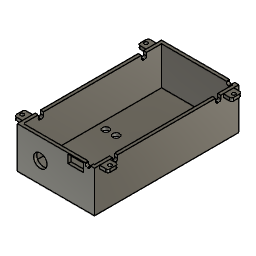
Cover_V3 (Autodesk Fusion 360 design; units mm, degrees)
part number: 2025-10-18-14-32-01-691
Autodesk Fusion 360 part; units mm, degrees
sketch "Sketch1" plane through (0, 0, 0) normal (0, 0, 1) x (1, 0, 0)
  line L0 (0, 0) -> (69, 0)
  line L1 (69, 0) -> (69, 140)
  line L2 (69, 140) -> (0, 140)
  line L3 (0, 140) -> (0, 0)
  line L4 (0, 140) -> (-3, 140)
  line L5 (-3, 140) -> (-3, 0)
  line L6 (-3, 0) -> (0, 0)
  line L7 (0, 0) -> (0, 140)
  line L8 (69, 140) -> (72, 140)
  line L9 (72, 140) -> (72, 0)
  line L10 (72, 0) -> (69, 0)
  line L11 (69, 0) -> (69, 140)
  line L12 (34.5, 140) -> (34.5, 0) construction
  line L13 (25, 0) -> (44, 0)
  line L14 (34.5, 2) -> (34.5, 0) construction
  circle A0 centre (8, 75) radius 3.275
  circle A1 centre (60, 60) radius 6
  circle A2 centre (18, 75) radius 3.275
  line L15 (1.1966, 84.5922) -> (38.7187, 84.5357) construction
  line L16 (38.7187, 84.5357) -> (38.7111, 79.5066) construction
  line L17 (38.7111, 79.5066) -> (1.189, 79.563) construction
  line L18 (1.189, 79.563) -> (1.1966, 84.5922) construction
  circle A3 centre (60, 40) radius 3.5
  line L19 (69, 3) -> (0, 3)
  line L20 (69, 137) -> (0, 137)
  circle A4 centre (77, 130) radius 1.7
  line L21 (72, 140) -> (112, 140) construction
  line L22 (72, 125) -> (78, 125)
  line L23 (80, 127) -> (80, 133)
  line L24 (78, 135) -> (72, 135)
  line L25 (72, 135) -> (72, 125)
  circle A5 centre (77, 10) radius 1.7
  line L26 (72, 0) -> (100, 0) construction
  line L27 (72, 5) -> (78, 5)
  line L28 (80, 7) -> (80, 13)
  line L29 (78, 15) -> (72, 15)
  line L30 (72, 15) -> (72, 5)
  circle A6 centre (-8, 10) radius 1.7
  line L31 (-3, 0) -> (-18, 0) construction
  line L32 (-3, 15) -> (-9, 15)
  line L33 (-11, 13) -> (-11, 7)
  line L34 (-9, 5) -> (-3, 5)
  line L35 (-3, 5) -> (-3, 15)
  line L36 (-3, 140) -> (-16, 140) construction
  circle A7 centre (-8, 130) radius 1.7
  line L37 (-3, 135) -> (-9, 135)
  line L38 (-11, 133) -> (-11, 127)
  line L39 (-9, 125) -> (-3, 125)
  line L40 (-3, 125) -> (-3, 135) construction
  arc A8 (-11, 127) -> (-9, 125) centre (-9, 127) ccw
  arc A9 (-9, 135) -> (-11, 133) centre (-9, 133) ccw
  arc A10 (-9, 15) -> (-11, 13) centre (-9, 13) ccw
  arc A11 (-11, 7) -> (-9, 5) centre (-9, 7) ccw
  arc A12 (80, 13) -> (78, 15) centre (78, 13) ccw
  arc A13 (78, 5) -> (80, 7) centre (78, 7) ccw
  arc A14 (78, 125) -> (80, 127) centre (78, 127) ccw
  arc A15 (80, 133) -> (78, 135) centre (78, 133) ccw
  point P0 (-11, 15)
  point P1 (-11, 135)
  dimension "d1" = 140
  dimension "d3" = 3
  dimension "d4" = 3
  dimension "d30" = 75
  dimension "d35" = 6.55
  dimension "d36" = 65
  dimension "d37" = 12
  dimension "d38" = 60
  dimension "d40" = 6.55
  dimension "d41" = 10
  dimension "d42" = 3.5
  dimension "d46" = 7
  dimension "d47" = 40
  dimension "d48" = 3
  dimension "d49" = 3
  dimension "d64" = 3.4
  dimension "d65" = 5
  dimension "d66" = 10
  dimension "d67" = 8
  dimension "d68" = 10
  dimension "d69" = 5
  dimension "d70" = 3.4
  dimension "d71" = 5
  dimension "d72" = 10
  dimension "d73" = 10
  dimension "d74" = 5
  dimension "d75" = 8
  dimension "d76" = 3.4
  dimension "d77" = 5
  dimension "d78" = 10
  dimension "d79" = 8
  dimension "d80" = 10
  dimension "d81" = 5
  dimension "d82" = 3.4
  dimension "d83" = 5
  dimension "d84" = 10
  dimension "d85" = 8
  dimension "d86" = 10
  dimension "d87" = 5
  dimension "d88" = 2
  dimension "d89" = 2
  dimension "d90" = 2
  dimension "d91" = 2
  dimension "d92" = 2
  dimension "d93" = 2
  dimension "d94" = 2
  dimension "d95" = 2
  text T0 "CELL GPS\n" font "Arial" height 3.5 align left top in box 37.5222 x 5.0292 at (1.1966, 84.5922) x (0.999999, -0.001504) y (-0.001504, -0.999999) spacing 1 kerned
  constraint horizontal L0
  constraint vertical L1
  constraint horizontal L2
  constraint vertical L3
  constraint coincident L0.start L3.end
  constraint horizontal L4
  constraint vertical L5
  constraint horizontal L6
  constraint vertical L7
  constraint horizontal L8
  constraint vertical L9
  constraint horizontal L10
  constraint vertical L11
  constraint midpoint L2 L12.start
  constraint midpoint L0 L12.end
  constraint horizontal L13
  constraint coincident L0 L13.start
  constraint midpoint L13 L12.end
  constraint coincident L12 L14.start
  constraint coincident L1 L19.start
  constraint coincident L3 L19.end
  constraint perpendicular L3 L19
  constraint coincident L1 L20.start
  constraint perpendicular L1 L20
  constraint perpendicular L9 L21
  constraint horizontal L22
  constraint vertical L23
  constraint horizontal L24
  constraint vertical L25
  constraint coincident L9 L22.start
  constraint perpendicular L9 L26
  constraint horizontal L27
  constraint vertical L28
  constraint horizontal L29
  constraint vertical L30
  constraint coincident L9 L27.start
  constraint perpendicular L5 L31
  constraint horizontal L32
  constraint vertical L33
  constraint horizontal L34
  constraint vertical L35
  constraint coincident L5 L32.start
  constraint perpendicular L5 L36
  constraint horizontal L37
  constraint vertical L38
  constraint horizontal L39
  constraint vertical L40
  constraint coincident L5 L37.start
  constraint tangent L38 A8
  constraint tangent L39 A8
  constraint coincident P1 L37
  constraint coincident P1 L38
  constraint tangent L37 A9
  constraint tangent L38 A9
  constraint coincident P0 L32
  constraint coincident P0 L33
  constraint tangent L32 A10
  constraint tangent L33 A10
  constraint tangent L33 A11
  constraint tangent L34 A11
  constraint tangent L28 A12
  constraint tangent L29 A12
  constraint tangent L27 A13
  constraint tangent L28 A13
  constraint tangent L22 A14
  constraint tangent L23 A14
  constraint tangent L23 A15
  constraint tangent L24 A15
  measures "d1" distance of L0.start L2.end
  measures "d3" distance of L5 L7
  measures "d4" distance of L9 L11
  measures "d30" distance of L5 L9
  measures "d35" diameter of A0
  measures "d36" distance of L2 A0.centre
  measures "d37" diameter of A1
  measures "d38" distance of L0 A1.centre
  measures "d40" diameter of A2
  measures "d41" distance of A0.centre A2.centre
  measures "d46" diameter of A3
  measures "d47" distance of L0 A3.centre
  measures "d48" distance of L13 L19
  measures "d49" distance of L2 L20
  measures "d64" diameter of A4
  measures "d65" distance of L9 A4.centre
  measures "d66" distance of A4.centre L21
  measures "d67" distance of L23 L25
  measures "d68" distance of L22 L24
  measures "d69" distance of L21 L24
  measures "d70" diameter of A5
  measures "d71" distance of L9 A5.centre
  measures "d72" distance of A5.centre L26
  measures "d73" distance of L27 L29
  measures "d74" distance of L26 L27
  measures "d75" distance of L9 L28
  measures "d76" diameter of A6
  measures "d77" distance of L5 A6.centre
  measures "d78" distance of A6.centre L31
  measures "d79" distance of L32.start P0
  measures "d80" distance of L32.start L34.end
  measures "d81" distance of L31 L34
  measures "d82" diameter of A7
  measures "d83" distance of L5 A7.centre
  measures "d84" distance of L36 A7.centre
  measures "d85" distance of L37.start P1
  measures "d86" distance of L37.start L39.end
  measures "d87" distance of L36 L37
  measures "d88" radius of A8
  measures "d89" radius of A9
  measures "d90" radius of A10
  measures "d91" radius of A11
  measures "d92" radius of A12
  measures "d93" radius of A13
  measures "d94" radius of A14
  measures "d95" radius of A15
extrude "Extrude1" add sketch "Sketch1" along normal blind 3 contours L0 L1 L3 L7 L11 L13 L19 | L1 L3 L7 L11 L19 L20 | L1 L2 L3 L7 L11 L20 makes body 1
extrude "Extrude2" add sketch "Sketch1" along normal blind 40 contours L0 L1 L3 L7 L11 L13 L19 | L3 L4 L5 L6 L7 L35 | L1 L2 L3 L7 L11 L20 | L1 L8 L9 L10 L11 L25 L30 bodies 1
sketch "Sketch3" plane through (72, 0, 0) normal (1, 0, 0) x (0, 1, 0)
  line L0 (0, 0) -> (140, 0)
  line L1 (140, 0) -> (140, 40)
  line L2 (140, 40) -> (0, 40)
  line L3 (0, 40) -> (0, 0)
  line L4 (140, 0) -> (0, 0)
  line L5 (70, 40) -> (70, 0) construction
  line L6 (17.5, 40) -> (22.5, 40)
  line L7 (22.5, 40) -> (22.5, 37)
  line L8 (20.5, 35) -> (19.5, 35)
  line L9 (17.5, 37) -> (17.5, 40)
  arc A0 (17.5, 37) -> (19.5, 35) centre (19.5, 37) ccw
  arc A1 (20.5, 35) -> (22.5, 37) centre (20.5, 37) ccw
  line L10 (20, 40) -> (20, 35) construction
  line L11 (117.5, 40) -> (122.5, 40)
  line L12 (122.5, 40) -> (122.5, 37)
  line L13 (120.5, 35) -> (119.5, 35)
  line L14 (117.5, 37) -> (117.5, 40)
  arc A2 (117.5, 37) -> (119.5, 35) centre (119.5, 37) ccw
  arc A3 (120.5, 35) -> (122.5, 37) centre (120.5, 37) ccw
  line L15 (120, 35) -> (120, 40) construction
  point P0 (17.5, 35)
  point P1 (117.5, 35)
  dimension "d18" = 5
  dimension "d19" = 5
  dimension "d20" = 2
  dimension "d21" = 2
  dimension "d23" = 5
  dimension "d24" = 2
  dimension "d25" = 2
  dimension "d26" = 5
  dimension "d27" = 100
  constraint midpoint L2 L5.start
  constraint midpoint L4 L5.end
  constraint horizontal L6
  constraint vertical L7
  constraint horizontal L8
  constraint vertical L9
  constraint coincident L2 L6.start
  constraint coincident P0 L8
  constraint coincident P0 L9
  constraint tangent L8 A0
  constraint tangent L9 A0
  constraint tangent L7 A1
  constraint tangent L8 A1
  constraint midpoint L6 L10.start
  constraint midpoint L8 L10.end
  constraint horizontal L11
  constraint vertical L12
  constraint horizontal L13
  constraint vertical L14
  constraint coincident L2 L11.start
  constraint coincident P1 L13
  constraint coincident P1 L14
  constraint tangent L13 A2
  constraint tangent L14 A2
  constraint tangent L12 A3
  constraint tangent L13 A3
  constraint midpoint L13 L15.start
  constraint midpoint L11 L15.end
  constraint symmetric L5 L10 L15
  measures "d18" distance of L6.start P0
  measures "d19" distance of L7 L9
  measures "d20" radius of A0
  measures "d21" radius of A1
  measures "d23" distance of L12 L14
  measures "d24" radius of A2
  measures "d25" radius of A3
  measures "d26" distance of L11 L13
  measures "d27" distance of L10 L15
extrude "Extrude3" cut sketch "Sketch3" along normal mid plane 200 contours L2 L6 L7 L8 L9 A0 A1 | L2 L11 L12 L13 L14 A2 A3 bodies 1
extrude "Extrude4" cut sketch "Sketch1" along normal blind 1 text T0 bodies 1
sketch "Sketch4" plane through (0, 0, 0) normal (0, -1, 0) x (1, 0, 0)
  line L0 (-3, 0) -> (72, 0)
  line L1 (72, 0) -> (72, 40)
  line L2 (72, 40) -> (-3, 40)
  line L3 (-3, 40) -> (-3, 0)
  line L4 (63, 40) -> (68, 40)
  line L5 (68, 40) -> (68, 39)
  line L6 (66, 37) -> (65, 37)
  line L7 (63, 39) -> (63, 40)
  arc A0 (63, 39) -> (65, 37) centre (65, 39) ccw
  arc A1 (66, 37) -> (68, 39) centre (66, 39) ccw
  line L8 (64.5, 9) -> (4.5, 9) construction
  line L9 (4.5, 9) -> (4.5, 31) construction
  line L10 (4.5, 31) -> (64.5, 31) construction
  line L11 (64.5, 31) -> (64.5, 9) construction
  line L12 (34.5, 0) -> (34.5, 40) construction
  line L13 (34.5, 9) -> (34.5, 31) construction
  line L14 (72, 20) -> (-3, 20) construction
  line L15 (4.5, 20) -> (64.5, 20) construction
  circle A2 centre (19.5, 20) radius 6.5
  line L16 (61.2478, 39) -> (46.2478, 39)
  line L17 (46.2478, 39) -> (46.2478, 31)
  line L18 (46.2478, 31) -> (61.2478, 31)
  line L19 (61.2478, 31) -> (61.2478, 39)
  dimension "d50" = 5
  dimension "d51" = 3
  dimension "d53" = 2
  dimension "d54" = 2
  dimension "d57" = 4
  dimension "d58" = 60
  dimension "d59" = 22
  dimension "d60" = 13
  dimension "d61" = 15
  dimension "d99" = 15
  dimension "d100" = 8
  dimension "d101" = 1
  constraint horizontal L4
  constraint vertical L5
  constraint horizontal L6
  constraint vertical L7
  constraint coincident L2 L4.start
  constraint tangent L6 A0
  constraint tangent L7 A0
  constraint tangent L5 A1
  constraint tangent L6 A1
  constraint horizontal L8
  constraint vertical L9
  constraint horizontal L10
  constraint vertical L11
  constraint midpoint L0 L12.start
  constraint midpoint L2 L12.end
  constraint midpoint L8 L13.start
  constraint midpoint L10 L13.end
  constraint collinear L12 L13
  constraint midpoint L1 L14.start
  constraint midpoint L3 L14.end
  constraint midpoint L9 L15.start
  constraint midpoint L11 L15.end
  constraint collinear L14 L15
  constraint coincident L14 A2.centre
  constraint horizontal L16
  constraint vertical L17
  constraint horizontal L18
  constraint vertical L19
  measures "d50" distance of L5 L7
  measures "d51" distance of L4 L6
  measures "d53" radius of A0
  measures "d54" radius of A1
  measures "d57" distance of L1.end L4.end
  measures "d58" distance of L8.start L8.end
  measures "d59" distance of L8.start L10.end
  measures "d60" diameter of A2
  measures "d61" distance of L9 A2.centre
  measures "d99" distance of L16.start L16.end
  measures "d100" distance of L16.start L18.end
  measures "d101" distance of L2 L16
extrude "Extrude5" cut sketch "Sketch4" against normal blind 200 contours L2 L4 L5 L6 L7 A0 A1 bodies 1
extrude "Extrude6" cut sketch "Sketch4" against normal blind 5 contours A2 | L16 L17 L18 L19 bodies 1
extrude "Extrude7" add sketch "Sketch1" along normal blind 3 from surface at 37 separate body contours L5 L32 L33 L34 L35 A10 A11 | L5 L37 L38 L39 A8 A9 | L9 L27 L28 L29 L30 A12 A13 | L9 L22 L23 L24 L25 A14 A15 makes body 2 at (73.1, 10, 37) makes body 3 at (-4.1, 130, 37) makes body 4 at (73.1, 130, 37) makes body 5 at (-4.1, 10, 37)
